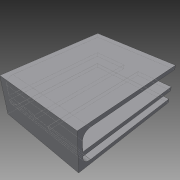
# Autodesk Inventor part: HanesBand-Adjuster
Saved by Autodesk Inventor 2015 (Build 190159000, 159)
## iProperties
Created: 2020-03-26
Part Number: HanesBand-Adjuster
Material: Generic
Document SubType Name: Modeling
Designer: Dominick Lee
Density: 1 g/cm^3
Appearance: Default
Author: Dominick Lee
Autodesk Inventor part; units mm, degrees
ref_plane "YZ Plane" through (0, 0, 0) normal (1, 0, 0) x (0, 1, 0)
ref_plane "XZ Plane" through (0, 0, 0) normal (0, 1, 0) x (-1, 0, 0)
ref_plane "XY Plane" through (0, 0, 0) normal (0, 0, 1) x (1, 0, 0)
sketch "Sketch1" plane through (0, 0, 0) normal (0, 1, 0) x (-1, 0, 0)
  line L0 (12.5, 5.5) -> (-12.5, 5.5)
  line L1 (-12.5, 5.5) -> (-12.5, -5.5)
  line L2 (-12.5, -5.5) -> (12.5, -5.5)
  line L3 (12.5, -5.5) -> (12.5, 5.5)
  line L4 (12.5, 5.5) -> (-12.5, -5.5) construction
  line L5 (-12.5, 5.5) -> (12.5, -5.5) construction
  point P0 (0, 0)
  dimension "d0" = 25
  dimension "d1" = 11
  constraints: 12 end point, 2 midpoint, 2 parallel, 1 horizontal, 1 perpendicular
  measures "d0" distance of L0.start L0.end
  measures "d1" distance of L1.end L0.end
extrude "Extrusion1" add sketch "Sketch1" along normal blind 1.2
sketch "Sketch2" plane through (0, 1.2, 0) normal (0, 1, 0) x (1, 0, 0)
  line L0 (-12.5, 5.5) -> (12.5, 5.5)
  line L1 (12.5, 5.5) -> (12.5, 4.3)
  line L2 (12.5, 4.3) -> (-12.5, 4.3)
  line L3 (-12.5, 4.3) -> (-12.5, 5.5)
  line L4 (0, 4.3) -> (0, 1.8)
  line L5 (-12.5, 5.5) -> (-12.5, -5.5) projected
  line L6 (-12.5, 5.5) -> (-12.5, -5.5) projected
  line L7 (0, 0.6) -> (0, -4.3)
  line L8 (-12.5, -4.3) -> (12.5, -4.3)
  line L9 (12.5, -5.5) -> (12.5, -4.3)
  line L10 (-12.5, -4.3) -> (-12.5, -5.5)
  line L11 (-12.5, -5.5) -> (12.5, -5.5)
  line L12 (-2.4, 1.7967) -> (-2.4, 0.6)
  line L13 (-2.4, 0.6) -> (2.4, 0.6)
  line L14 (2.4, 0.6) -> (2.4, 1.7967)
  line L15 (-2.4, 1.7967) -> (2.4, 0.6) construction
  line L16 (-2.4, 0.6) -> (2.4, 1.7967) construction
  line L17 (-2.4, 1.7967) -> (-12.5, 1.7967)
  line L18 (-12.5, 0.6) -> (-12.5, 1.7967)
  line L19 (-12.5, 0.6) -> (-2.4, 0.6)
  line L20 (2.4, 1.7967) -> (12.5, 1.7967)
  line L21 (12.5, -5.5) -> (12.5, 5.5) projected
  line L22 (2.4, 0.6) -> (12.5, 0.6)
  line L23 (12.5, 0.6) -> (12.5, 1.7967)
  point P0 (0, 0)
  point P1 (0, 1.1983)
  dimension "d4" = 1.2
  dimension "d5" = 2.5
  dimension "d7" = 4.9
  dimension "d11" = 4.8
  constraints: 42 end point, 8 vertical, 7 point on line, 6 horizontal, 3 midpoint, 1 parallel, 1 perpendicular
  measures "d4" distance of L0.end L1.end
  measures "d5" distance of L4.start L4.end
  measures "d7" distance of L7.start L7.end
  measures "d11" distance of L13.end L12.end
extrude "Extrusion2" add sketch "Sketch2" along normal blind 30 contours L0 L1 L2 L3 | L17 L12 L19 L5 | L21 L22 L14 L20 | L8 L9 L11 L5
fillet "Fillet1" radius 2 2 edges at (0, 1.2, 4.3) (0, 1.2, -4.3)
body "Solid1"
